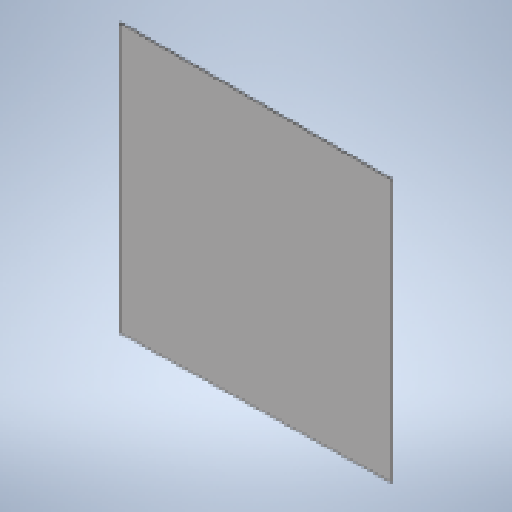
# Autodesk Inventor part: GBK 2311 shield 7
Saved by Autodesk Inventor 2026 (Build 300175000, 175)
## iProperties
Created: 2026-04-17
Part Number: GBK 2311 shield 7
Material: Steel
Document SubType Name: Sheet Metal
Designer: pokla
Stock Number: 2317
Mass: 69243.3 g
Surface Area: 44341.6 cm^2
Volume: 8820.8 cm^3
Density: 7.85 g/cm^3
Flat Pattern Width: 148 cm
Flat Pattern Length: 146.3 cm
Flat Pattern Area: 21652.4 cm^2
Sheet Metal Rule: По умолчанию_мм
Sheet Metal Width: 1480,000 мм
Sheet Metal Length: 1463,000 мм
Sheet Metal Area: 2165240,000 мм^2
Appearance: Default
Author: admin
Autodesk Inventor part; units mm, degrees
ref_plane "YZ Plane" through (0, 0, 0) normal (1, 0, 0) x (0, 1, 0)
ref_plane "XZ Plane" through (0, 0, 0) normal (0, 1, 0) x (-1, 0, 0)
ref_plane "XY Plane" through (0, 0, 0) normal (0, 0, 1) x (1, 0, 0)
sketch "Sketch1" plane through (0, 0, 0) normal (0, 0, 1) x (1, 0, 0)
  line L0 (740, -745) -> (-740, -745)
  line L1 (-740, -745) -> (-740, 745)
  line L2 (-740, 745) -> (740, 745)
  line L3 (740, 745) -> (740, -745)
  line L4 (740, -745) -> (-740, 745) construction
  line L5 (-740, -745) -> (740, 745) construction
  line L6 (-740, -718) -> (740, -684.4141)
  point P0 (0, 0)
  point P1 (740, -711.4141)
  dimension "d0" = 1480
  dimension "d1" = 1490
  dimension "d4" = 1.3
  dimension "d5" = 27
  measures "d0" distance of L1.end L2.end
  measures "d1" distance of L0.end L1.end
  measures "d4" angle of L0 L6
  measures "d5" distance of L0.end L6.start
extrude "Plate1" add sketch "Sketch1" along normal blind 4 contours L6 L1 L2 L3
sketch "Эскиз3" plane through (0, 0, 0) normal (0, 0, -1) x (-1, 0, 0)
  line L0 (565.9636, -544.2731) -> (565.9636, -1042.4092) construction
  line L1 (565.9636, -1042.4092) -> (526.3364, -1042.4092) construction
  line L2 (526.3364, -1042.4092) -> (526.3364, -544.2731) construction
  line L3 (526.3364, -544.2731) -> (565.9636, -544.2731) construction
  line L4 (710, -491) -> (710, -487) construction
  line L5 (710, 5.6667) -> (710, 9.6667) construction
  line L6 (710, -491) -> (710, -487) projected
  line L7 (710, 5.6667) -> (710, 9.6667) projected
  line L8 (710, 502.3333) -> (710, 506.3333) projected
  line L9 (230.5109, -494.5) -> (230.5109, -591.5) projected
  line L10 (230.5109, -591.5) -> (226.5119, -591.5) projected
  line L11 (-269.6177, -494.5) -> (-269.6177, -591.5) projected
  line L12 (-269.6177, -591.5) -> (-273.6167, -591.5) projected
  line L13 (-739.3197, -491) -> (-710, -491) projected
  line L14 (-710, -491) -> (-710, -487) projected
  line L15 (-739.3197, 5.6667) -> (-710, 5.6667) projected
  line L16 (-710, 5.6667) -> (-710, 9.6667) projected
  line L17 (-739.3197, 502.3333) -> (-710, 502.3333) projected
  line L18 (-710, 502.3333) -> (-710, 506.3333) projected
  ellipse E0 centre (-269.6177, 743.5) end of major axis (-269.6177, 773.5) minor radius 0.6803 (-269.6177, 713.5) -> (-269.6177, 773.5) ccw projected
  line L19 (-269.6177, 713.5) -> (-273.6167, 713.5) projected
  ellipse E1 centre (230.5109, 743.5) end of major axis (230.5109, 773.5) minor radius 0.6803 (230.5109, 713.5) -> (230.5109, 773.5) ccw projected
  line L20 (230.5109, 713.5) -> (226.5119, 713.5) projected
  point P0 (0, 0)
  constraints: 4 other
mark "Маркировка1"
equation "\"d0\" = Лист_ширина"
equation "\"d2\" = Thickness"
equation "\"BendRadius\" = Thickness"
equation "\"BendReliefWidth\" = Thickness"
equation "\"BendReliefDepth\" = 0.5 * Thickness"
equation "\"CornerReliefSize\" = 4 * Thickness"
equation "\"MinimumRemnant\" = 2 * Thickness"
equation "\"TransitionRadius\" = BendRadius"
equation "\"JacobiRadiusSize\" = BendRadius"
equation "\"GapSize\" = Thickness"
equation "\"Лист_ширина\" = 1480"
equation "\"Thickness\" = 4"
body "Solid1"
